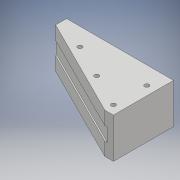
# Autodesk Inventor part: wrist adapter
Saved by Autodesk Inventor 2017 (Build 210142000, 142)
## iProperties
Created: 2018-02-13
Part Number: wrist adapter
Material: Generic
Document SubType Name: Modeling
Designer: JT
Density: 1 g/cm^3
Appearance: Default
Author: JT
Autodesk Inventor part; units mm, degrees
ref_plane "YZ Plane" through (0, 0, 0) normal (1, 0, 0) x (0, 1, 0)
ref_plane "XZ Plane" through (0, 0, 0) normal (0, 1, 0) x (-1, 0, 0)
sketch "Sketch2" plane through (0, 0, 0) normal (0, 0, 1) x (1, 0, 0)
  line L0 (20, -8) -> (-10, -8) construction
  line L1 (-10, -8) -> (-10, -23) construction
  line L2 (-10, -23) -> (20, -23) construction
  line L3 (20, -23) -> (20, -8) construction
  line L4 (20, -8) -> (-10, -23) construction
  line L5 (-10, -8) -> (20, -23) construction
  point P0 (5, -15.5)
  point P1 (5, -15.5)
  point P2 (0, 0)
  dimension "d2" = 30
  dimension "d3" = 15
  dimension "d4" = 5
  dimension "d5" = 8
  constraints: 12 end point, 4 coincident, 2 midpoint, 2 parallel, 1 horizontal, 1 perpendicular
  measures "d2" distance of L2.end L1.end
  measures "d3" distance of L1.end L0.end
  measures "d4" horizontal distance of point (5, -15.5) point (0, 0)
  measures "d5" distance from line of point (0, 0) L0
sketch "Sketch3" plane through (0, 0, 0) normal (0, 0, 1) x (1, 0, 0)
  line L0 (24, 0) -> (24, -27)
  line L1 (24, -27) -> (20.1738, -27)
  line L2 (20.1738, -27) -> (-24, -4.9131)
  line L3 (-24, -4.9131) -> (-24, 0)
  line L4 (-24, 0) -> (24, 0)
  line L5 (20, -23) -> (-10, -8) construction
  point P0 (0, 0)
  point P1 (5, -15.5)
  point P2 (20, -8)
  dimension "d6" = 4
  dimension "d8" = 3.5
  dimension "d9" = 4
  constraints: 12 end point, 2 midpoint, 2 parallel, 2 perpendicular, 1 vertical
  measures "d6" distance from line of L5.start L0
  measures "d8" distance between parallel lines of L2 L5
  measures "d9" distance from line of L5.start L1
extrude "Extrusion1" add sketch "Sketch3" along normal mid plane 18
sketch "Sketch4" plane through (0, 0, 9) normal (0, 0, 1) x (1, 0, 0)
  point P0 (0, 0)
  point P1 (20, -23)
  point P2 (5, -15.5)
  point P3 (-10, -8)
  point P4 (20, -8)
hole "Hole1" at (20, -23, 9) at (5, -15.5, 9) at (-10, -8, 9) at (20, -8, 9) direction (0, 0, -1) diameter 2 end through all
ref_plane "Work Plane1" through (21.5154, -24.3167, -9) normal (-0.4472, -0.8944, 0) x (0.8944, -0.4472, 0)
sketch "Sketch9" plane through (20.1738, -27, -9) normal (-0.4472, -0.8944, 0) x (0.8944, -0.4472, 0)
  line L0 (19.8813, 12) -> (-80.1187, 12)
  line L1 (-80.1187, 12) -> (-80.1187, 6)
  line L2 (-80.1187, 6) -> (19.8813, 6)
  line L3 (19.8813, 6) -> (19.8813, 12)
  line L4 (19.8813, 12) -> (-80.1187, 6) construction
  line L5 (-80.1187, 12) -> (19.8813, 6) construction
  point P0 (-30.1187, 9)
  dimension "d54" = 6
  dimension "d55" = 100
  constraints: 12 end point, 2 midpoint, 2 parallel, 1 horizontal, 1 perpendicular
  measures "d54" distance between parallel lines of L0 L2
  measures "d55" distance between parallel lines of L1 L3
extrude "Extrusion2" cut sketch "Sketch9" against normal blind 0.5
sketch "Sketch10" plane through (-24, 0, 9) normal (0, 1, 0) x (1, 0, 0)
  line L0 (24, 9) -> (42.9051, 9) construction
  point P0 (24, 13.5)
  point P1 (24, 4.5)
  point P2 (10, 13.5)
  point P3 (10, 4.5)
  point P4 (38, 4.5)
  point P5 (38, 13.5)
  dimension "d58" = 9
  dimension "d59" = 14
  dimension "d60" = 14
  constraints: 4 horizontal alignment, 3 vertical alignment, 2 end point, 1 horizontal, 1 symmetric about line
  measures "d58" distance of point (24, 4.5) point (24, 13.5)
  measures "d59" distance of point (24, 13.5) point (10, 13.5)
  measures "d60" distance of point (38, 13.5) point (24, 13.5)
hole "Hole6" at (0, 0, -4.5) at (0, 0, 4.5) at (-14, 0, -4.5) at (-14, 0, 4.5) at (14, 0, 4.5) at (14, 0, -4.5) direction (0, -1, 0) diameter 3 depth 8 tip angle 118
body "Solid1"
